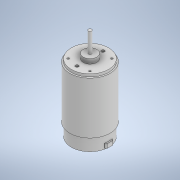
# Autodesk Inventor part: motor_1
Saved by Autodesk Inventor 2020 (Build 240168000, 168)
## iProperties
Created: 2019-04-23
Part Number: motor_1
Material: Generic
Document SubType Name: Modeling
Designer: psrob
Density: 1 g/cm^3
Appearance: Default
Author: psrob
Autodesk Inventor part; units mm, degrees
ref_plane "YZ Plane" through (0, 0, 0) normal (1, 0, 0) x (0, 1, 0)
ref_plane "XZ Plane" through (0, 0, 0) normal (0, 1, 0) x (-1, 0, 0)
sketch "Sketch1" plane through (0, 0, 0) normal (0, 1, 0) x (-1, 0, 0)
  circle A0 centre (0, 0) radius 18
  dimension "d0" = 36
  constraints: 1 centre point, 1 coincident
  measures "d0" diameter of A0
extrude "Extrusion1" add sketch "Sketch1" along normal blind 65
ref_plane "Work Plane1" through (0, 62.4, 0) normal (0, 1, 0) x (1, 0, 0)
sketch "Sketch2" plane through (0, 62.4, 0) normal (0, 1, 0) x (1, 0, 0)
  circle A0 centre (0, 0) radius 18 projected
  circle A1 centre (0, 0) radius 19.4
  line L0 (-15.5, -1.35) -> (-20.5, -1.35)
  line L1 (-20.5, -1.35) -> (-20.5, 1.35)
  line L2 (-20.5, 1.35) -> (-15.5, 1.35)
  line L3 (-15.5, 1.35) -> (-15.5, -1.35)
  circle A2 centre (0, 0) radius 18 projected
  line L4 (-15.5, -1.35) -> (-20.5, 1.35) construction
  line L5 (-20.5, -1.35) -> (-15.5, 1.35) construction
  point P0 (-18, 0)
  point P1 (-19.353, 1.35)
  point P2 (-17.9493, 1.35)
  point P3 (-17.9493, -1.35)
  point P4 (-19.353, -1.35)
  dimension "d4" = 38.8
  dimension "d5" = 5
  dimension "d6" = 2.7
  constraints: 12 end point, 2 midpoint, 2 parallel, 1 centre point, 1 coincident, 1 horizontal, 1 horizontal alignment, 1 perpendicular, 1 other
  measures "d4" diameter of A1
  measures "d5" distance of L1.end L2.end
  measures "d6" distance of L0.end L1.end
extrude "Extrusion2" add sketch "Sketch2" against normal blind 50 contours A0 L2 A1 L0 picked at (18.5875, 2.9161)
sketch "Sketch3" plane through (0, 65, 0) normal (0, 1, 0) x (1, 0, 0)
  circle A0 centre (0, 0) radius 18 projected
  circle A1 centre (0, 0) radius 6.5
  dimension "d9" = 13
  constraints: 1 centre point, 1 coincident
  measures "d9" diameter of A1
extrude "Extrusion3" add sketch "Sketch3" along normal blind 4.5 contours A1
sketch "Sketch4" plane through (0, 0, 0) normal (0, -1, 0) x (1, 0, 0)
  circle A0 centre (0, 0) radius 18 projected
  circle A1 centre (0, 0) radius 5.1
  dimension "d12" = 10.2
  constraints: 1 centre point, 1 coincident
  measures "d12" diameter of A1
extrude "Extrusion4" add sketch "Sketch4" along normal blind 3.4 contours A1
sketch "Sketch5" plane through (0, 65, 0) normal (0, 1, 0) x (1, 0, 0)
  circle A0 centre (0, 0) radius 6.5 projected
  circle A1 centre (0, 0) radius 18 projected
  line L0 (0, 0) -> (0, -12.5)
  line L1 (0, 0) -> (0, 12.5)
  circle A2 centre (0, -12.5) radius 1.5
  circle A3 centre (0, 12.5) radius 1.5
  dimension "d15" = 12.5
  dimension "d16" = 12.5
  dimension "d17" = 3
  dimension "d18" = 3
  constraints: 4 end point, 2 centre point, 2 coincident, 2 vertical
  measures "d15" distance of L0.start L0.end
  measures "d16" distance of L0.start L1.end
  measures "d17" diameter of A2
  measures "d18" diameter of A3
extrude "Extrusion5" cut sketch "Sketch5" against normal blind 3 contours A2 | A3
sketch "Sketch6" plane through (0, 65, 0) normal (0, 1, 0) x (1, 0, 0)
  circle A0 centre (0, 0) radius 6.5 projected
  line L0 (10.5, 10.5) -> (-10.5, 10.5)
  line L1 (-10.5, 10.5) -> (-10.5, -10.5)
  line L2 (-10.5, -10.5) -> (10.5, -10.5)
  line L3 (10.5, -10.5) -> (10.5, 10.5)
  circle A1 centre (0, 0) radius 5.1 projected
  line L4 (10.5, 10.5) -> (-10.5, -10.5) construction
  line L5 (-10.5, 10.5) -> (10.5, -10.5) construction
  circle A2 centre (10.5, -10.5) radius 1
  circle A3 centre (-10.5, -10.5) radius 1
  circle A4 centre (-10.5, 10.5) radius 1
  circle A5 centre (10.5, 10.5) radius 1
  dimension "d21" = 21
  dimension "d22" = 21
  dimension "d23" = 2
  dimension "d24" = 2
  dimension "d25" = 2
  dimension "d26" = 2
  constraints: 12 end point, 4 centre point, 4 coincident, 2 midpoint, 2 parallel, 1 horizontal, 1 perpendicular
  measures "d21" distance of L2.end L1.end
  measures "d22" distance of L0.end L1.end
  measures "d23" diameter of A2
  measures "d24" diameter of A3
  measures "d25" diameter of A4
  measures "d26" diameter of A5
extrude "Extrusion6" cut sketch "Sketch6" against normal blind 1 contours A4 L1 L0 | L0 L1 A4 | A5 L3 L0 | L0 L3 A5 | A3 L2 L1 | L1 L2 A3 | A2 L2 L3 | L3 L2 A2
sketch "Sketch7" plane through (0, 65, 0) normal (0, 1, 0) x (1, 0, 0)
  circle A0 centre (0, 0) radius 6.5 projected
  circle A1 centre (0, 0) radius 1.5875
  dimension "d29" = 3.175
  constraints: 1 centre point, 1 coincident
  measures "d29" diameter of A1
extrude "Extrusion7" add sketch "Sketch7" against normal blind 76.2 contours A1
sketch "Sketch8" plane through (0, -11.2, 0) normal (0, -1, 0) x (1, 0, 0)
  circle A0 centre (0, 0) radius 1.5875 projected
extrude "Extrusion8" add sketch "Sketch8" against normal blind 100
sketch "Sketch9" plane through (0, 0, 0) normal (0, -1, 0) x (1, 0, 0)
  circle A0 centre (0, 0) radius 5.1 projected
  circle A1 centre (0, 0) radius 18 projected
  circle A2 centre (0, 0) radius 1.5875 projected
  line L0 (0, 0) -> (19.2, 0)
  line L1 (16.8, -3.75) -> (19.2, -3.75)
  line L2 (19.2, -3.75) -> (19.2, 3.75)
  line L3 (19.2, 3.75) -> (16.8, 3.75)
  line L4 (16.8, 3.75) -> (16.8, -3.75)
  circle A3 centre (0, 0) radius 18 projected
  line L5 (16.8, -3.75) -> (19.2, 3.75) construction
  line L6 (19.2, -3.75) -> (16.8, 3.75) construction
  point P0 (18, 0)
  dimension "d34" = 19.2
  dimension "d35" = 2.4
  dimension "d36" = 7.5
  constraints: 14 end point, 2 horizontal, 2 midpoint, 2 parallel, 1 horizontal alignment, 1 perpendicular, 1 point on line, 1 other
  measures "d34" distance of L0.start L0.end
  measures "d35" distance of L3.end L2.end
  measures "d36" distance of L2.end L1.end
extrude "Extrusion9" add sketch "Sketch9" against normal blind 5 contours L4 L3 A1 L0 | L0 A1 L1 L4 | L0 L2 L1 A1 | A1 L3 L2 L0
chamfer "Chamfer1" distance 1 angle 45 2 edges at (19.2, 2.5, -3.75) (19.2, 2.5, 3.75)
sketch "Sketch10" plane through (0, 0, 0) normal (0, -1, 0) x (1, 0, 0)
  line L0 (19.2, 2.75) -> (18.2, 3.75) projected
  line L1 (19.2, 2.75) -> (19.2, -2.75) projected
  line L2 (18.2, -3.75) -> (19.2, -2.75) projected
  line L3 (18.2, -3.75) -> (17.605, -3.75) projected
  arc A0 (17.605, -3.75) -> (17.605, 3.75) centre (0, 0) ccw projected
  line L4 (17.605, 3.75) -> (18.2, 3.75) projected
extrude "Extrusion10" cut sketch "Sketch10" against normal blind 1
body "Solid1"
